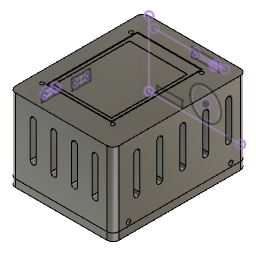
enviro-feather-box (Autodesk Fusion 360 design; units mm, degrees)
Autodesk Fusion 360 part; units mm, degrees
(part 1 of 2)
sketch "PCB" plane through (0, 0, 0) normal (0, 0, 1) x (1, 0, 0) in component "Feather HUZZAH ESP8266 v1"
  line L0 (0, 0) -> (50.8, 0)
  line L1 (50.8, 0) -> (50.8, -22.86)
  line L2 (50.8, -22.86) -> (0, -22.86)
  line L3 (0, -22.86) -> (0, 0)
  circle A0 centre (2.54, -20.32) radius 1.27
  circle A1 centre (2.54, -2.54) radius 1.27
  circle A2 centre (48.26, -21.0185) radius 1.145
  circle A3 centre (48.26, -1.905) radius 1.145
  dimension "d1_2" = 50.8
  dimension "d2_2" = 22.86
  dimension "d3_2" = 2.54
  dimension "d4_1" = 2.54
  dimension "d5_2" = 2.54
  dimension "d6_2" = 2.54
  dimension "d7_2" = 20.32
  dimension "d8_2" = 2.54
  dimension "d9_2" = 2.29
  dimension "d10_2" = 48.26
  dimension "d11_2" = 1.8415
  dimension "d12_2" = 2.29
  dimension "d13_2" = 20.955
  dimension "d14_1" = 48.26
  constraint horizontal L0
  constraint vertical L1
  constraint horizontal L2
  constraint vertical L3
  constraint coincident L0.start L3.end
  measures "d1_2" distance of L0.start L0.end
  measures "d2_2" distance of L0.start L2.end
  measures "d3_2" diameter of A0
  measures "d4_1" distance of L3 A0.centre
  measures "d5_2" distance of L2 A0.centre
  measures "d6_2" diameter of A1
  measures "d7_2" distance of L2 A1.centre
  measures "d8_2" distance of L3 A1.centre
  measures "d9_2" diameter of A2
  measures "d10_2" distance of L3 A2.centre
  measures "d11_2" distance of L2 A2.centre
  measures "d12_2" diameter of A3
  measures "d13_2" distance of L2 A3.centre
  measures "d14_1" distance of L3 A3.centre
extrude "Extrude1" add sketch "PCB" along normal blind 1.6 makes body 1 in component "Feather HUZZAH ESP8266 v1"
fillet "Fillet1" radius 2.54 4 edges at (0, -22.86, 0.8) (50.8, -22.86, 0.8) (50.8, 0, 0.8) (0, 0, 0.8) on bodies 1 in component "Feather HUZZAH ESP8266 v1"
sketch "usb" plane through (0, 0, 1.6) normal (0, 0, 1) x (-1, 0, 0) in component "Feather HUZZAH ESP8266 v1"
  circle A0 centre (-2.54, 20.32) radius 1.27
  circle A1 centre (-2.54, 2.54) radius 1.27
  circle A2 centre (-48.26, 21.0185) radius 1.145
  circle A3 centre (-48.26, 1.905) radius 1.145
  arc A4 (-2.54, 0) -> (0, 2.54) centre (-2.54, 2.54) ccw
  line L0 (0, 2.54) -> (0, 20.32)
  arc A5 (0, 20.32) -> (-2.54, 22.86) centre (-2.54, 20.32) ccw
  line L1 (-2.54, 22.86) -> (-48.26, 22.86)
  arc A6 (-48.26, 22.86) -> (-50.8, 20.32) centre (-48.26, 20.32) ccw
  line L2 (-50.8, 20.32) -> (-50.8, 2.54)
  arc A7 (-50.8, 2.54) -> (-48.26, 0) centre (-48.26, 2.54) ccw
  line L3 (-48.26, 0) -> (-2.54, 0)
  line L4 (0, 11.43) -> (-50.8, 11.43) construction
  line L5 (0, 15.33) -> (-5.6, 15.33)
  line L6 (-5.6, 15.33) -> (-5.6, 7.53)
  line L7 (-5.6, 7.53) -> (0, 7.53)
  line L8 (0, 7.53) -> (0, 15.33)
  line L9 (0, 15.33) -> (-5.6, 7.53) construction
  line L10 (-5.6, 15.33) -> (0, 7.53) construction
  point P0 (-2.8, 11.43)
  dimension "d18_1" = 7.8
  dimension "d19_1" = 5.6
  constraint midpoint L0 L4.start
  constraint midpoint L2 L4.end
  constraint perpendicular L5 L6
  constraint parallel L5 L7
  constraint parallel L6 L8
  constraint horizontal L5
  constraint coincident L9 P0
  constraint coincident L10 P0
  constraint coincident L4 P0
  constraint collinear L0 L8
  measures "d18_1" distance of L5.end L6.end
  measures "d19_1" distance of L6.end L7.end
extrude "Extrude2" add sketch "usb" along normal blind 2.95 separate body contours L0 L5 L6 L7 L8 makes body 2 in component "Feather HUZZAH ESP8266 v1"
chamfer "Chamfer1" distance 1 angle 45 2 edges at (2.8, -7.53, 1.6) (2.8, -15.33, 1.6) on bodies 2 in component "Feather HUZZAH ESP8266 v1"
sketch "modules" plane through (0, 0, 1.6) normal (0, 0, 1) x (-1, 0, 0) in component "Feather HUZZAH ESP8266 v1"
  circle A0 centre (-2.54, 20.32) radius 1.27
  circle A1 centre (-2.54, 2.54) radius 1.27
  circle A2 centre (-48.26, 21.0185) radius 1.145
  circle A3 centre (-48.26, 1.905) radius 1.145
  arc A4 (-2.54, 0) -> (0, 2.54) centre (-2.54, 2.54) ccw
  line L0 (0, 2.54) -> (0, 20.32)
  arc A5 (0, 20.32) -> (-2.54, 22.86) centre (-2.54, 20.32) ccw
  line L1 (-2.54, 22.86) -> (-48.26, 22.86)
  arc A6 (-48.26, 22.86) -> (-50.8, 20.32) centre (-48.26, 20.32) ccw
  line L2 (-50.8, 20.32) -> (-50.8, 2.54)
  arc A7 (-50.8, 2.54) -> (-48.26, 0) centre (-48.26, 2.54) ccw
  line L3 (-48.26, 0) -> (-2.54, 0)
  line L4 (-50.8, 11.43) -> (0, 11.43) construction
  line L5 (-26.8, 19.43) -> (-50.8, 19.43)
  line L6 (-50.8, 19.43) -> (-50.8, 3.43)
  line L7 (-50.8, 3.43) -> (-26.8, 3.43)
  line L8 (-26.8, 3.43) -> (-26.8, 19.43)
  line L9 (-26.8, 19.43) -> (-50.8, 3.43) construction
  line L10 (-50.8, 19.43) -> (-26.8, 3.43) construction
  line L11 (-28.4, 17.58) -> (-43.7, 17.58)
  line L12 (-43.7, 17.58) -> (-43.7, 5.28)
  line L13 (-43.7, 5.28) -> (-28.4, 5.28)
  line L14 (-28.4, 5.28) -> (-28.4, 17.58)
  line L15 (-28.4, 17.58) -> (-43.7, 5.28) construction
  line L16 (-43.7, 17.58) -> (-28.4, 5.28) construction
  point P0 (-38.8, 11.43)
  point P1 (-36.05, 11.43)
  dimension "d23_1" = 24
  dimension "d24_1" = 16
  dimension "d25_1" = 15.3
  dimension "d26_1" = 12.3
  dimension "d32_1" = 1.6
  constraint midpoint L2 L4.start
  constraint midpoint L0 L4.end
  constraint perpendicular L5 L6
  constraint parallel L5 L7
  constraint parallel L6 L8
  constraint horizontal L5
  constraint coincident L9 P0
  constraint coincident L10 P0
  constraint coincident L4 P0
  constraint perpendicular L11 L12
  constraint parallel L11 L13
  constraint parallel L12 L14
  constraint horizontal L11
  constraint coincident L15 P1
  constraint coincident L16 P1
  constraint coincident L4 P1
  measures "d23_1" distance of L6.end L7.end
  measures "d24_1" distance of L5.end L6.end
  measures "d25_1" distance of L12.end L13.end
  measures "d26_1" distance of L11.end L12.end
  measures "d32_1" distance of L8 L14
extrude "Extrude3" add sketch "modules" along normal blind 1 separate body contours L2 L5 L6 L7 L8 | L11 L12 L13 L14 makes body 3 in component "Feather HUZZAH ESP8266 v1"
extrude "Extrude4" add sketch "modules" along normal blind 2.4 and the other way blind -1 separate body contours L11 L12 L13 L14 makes body 4 in component "Feather HUZZAH ESP8266 v1"
sketch "JST" plane through (0, 0, 1.6) normal (0, 0, 1) x (-1, 0, 0) in component "Feather HUZZAH ESP8266 v1"
  circle A0 centre (-2.54, 20.32) radius 1.27
  circle A1 centre (-2.54, 2.54) radius 1.27
  circle A2 centre (-48.26, 21.0185) radius 1.145
  circle A3 centre (-48.26, 1.905) radius 1.145
  arc A4 (-2.54, 0) -> (0, 2.54) centre (-2.54, 2.54) ccw
  line L0 (0, 2.54) -> (0, 20.32)
  arc A5 (0, 20.32) -> (-2.54, 22.86) centre (-2.54, 20.32) ccw
  line L1 (-2.54, 22.86) -> (-48.26, 22.86)
  arc A6 (-48.26, 22.86) -> (-50.8, 20.32) centre (-48.26, 20.32) ccw
  line L2 (-50.8, 20.32) -> (-50.8, 2.54)
  arc A7 (-50.8, 2.54) -> (-48.26, 0) centre (-48.26, 2.54) ccw
  line L3 (-48.26, 0) -> (-2.54, 0)
  line L4 (-6.8, 0) -> (-14.8, 0)
  line L5 (-14.8, 0) -> (-14.8, 6)
  line L6 (-14.8, 6) -> (-6.8, 6)
  line L7 (-6.8, 6) -> (-6.8, 0)
  line L8 (-10.8, 0) -> (-10.8, 6) construction
  dimension "d33_1" = 8
  dimension "d34_1" = 6
  dimension "d35_1" = 10.8
  constraint horizontal L4
  constraint vertical L5
  constraint horizontal L6
  constraint vertical L7
  constraint midpoint L4 L8.start
  constraint midpoint L6 L8.end
  constraint collinear L3 L4
  measures "d33_1" distance of L4.start L4.end
  measures "d34_1" distance of L4.start L6.end
  measures "d35_1" distance of L0 L8
extrude "Extrude5" add sketch "JST" along normal blind 5.6 separate body contours L3 L4 L5 L6 L7 makes body 5 in component "Feather HUZZAH ESP8266 v1"
sketch "headers" plane through (0, 0, 1.6) normal (0, 0, 1) x (-1, 0, 0) in component "Feather HUZZAH ESP8266 v1"
  circle A0 centre (-48.26, 21.0185) radius 1.145
  circle A1 centre (-2.54, 2.54) radius 1.27
  circle A2 centre (-48.26, 1.905) radius 1.145
  circle A3 centre (-2.54, 20.32) radius 1.27
  arc A4 (-2.54, 0) -> (0, 2.54) centre (-2.54, 2.54) ccw
  line L0 (0, 2.54) -> (0, 20.32)
  arc A5 (0, 20.32) -> (-2.54, 22.86) centre (-2.54, 20.32) ccw
  line L1 (-2.54, 22.86) -> (-48.26, 22.86)
  arc A6 (-48.26, 22.86) -> (-50.8, 20.32) centre (-48.26, 20.32) ccw
  line L2 (-50.8, 20.32) -> (-50.8, 2.54)
  arc A7 (-50.8, 2.54) -> (-48.26, 0) centre (-48.26, 2.54) ccw
  line L3 (-48.26, 0) -> (-2.54, 0)
  line L4 (-15, 0) -> (-45.8, 0)
  line L5 (-45.8, 0) -> (-45.8, 2.6)
  line L6 (-45.8, 2.6) -> (-15, 2.6)
  line L7 (-15, 2.6) -> (-15, 0)
  line L8 (-6.2, 20.36) -> (-44.8, 20.36)
  line L9 (-44.8, 20.36) -> (-44.8, 22.86)
  line L10 (-44.8, 22.86) -> (-6.2, 22.86)
  line L11 (-6.2, 22.86) -> (-6.2, 20.36)
  dimension "d39_1" = 30.8
  dimension "d40_1" = 2.6
  dimension "d42_1" = 5
  dimension "d45_1" = 38.6
  dimension "d46_1" = 2.5
  dimension "d48_1" = 6
  constraint horizontal L4
  constraint vertical L5
  constraint horizontal L6
  constraint vertical L7
  constraint horizontal L8
  constraint vertical L9
  constraint horizontal L10
  constraint vertical L11
  constraint collinear L3 L4
  constraint collinear L1 L10
  measures "d39_1" distance of L4.start L4.end
  measures "d40_1" distance of L4.start L6.end
  measures "d42_1" distance of L2 L5
  measures "d45_1" distance of L8.start L8.end
  measures "d46_1" distance of L8.start L10.end
  measures "d48_1" distance of L2 L9
extrude "Extrude6" add sketch "headers" along normal blind 2.5 separate body contours L3 L4 L5 L6 L7 | L1 L8 L9 L10 L11 makes body 6 at (25.2667, -1.7333, 1.6) makes body 7 at (31.9333, -22.0267, 1.6) in component "Feather HUZZAH ESP8266 v1"
move_body "Move1" bodies 7 6 to x (1, 0, 0) y (0, 1, 0) z (0, 0, 1) at (0, 0, -4.1) in component "Feather HUZZAH ESP8266 v1"
sketch "pcb" plane through (0, 0, 0) normal (0, 0, 1) x (1, 0, 0) in component "2.4\" TFT Feather Wing Copy v1"
  line L0 (0, 0) -> (64.77, 0)
  line L1 (64.77, 0) -> (64.77, 52.578)
  line L2 (64.77, 52.578) -> (0, 52.578)
  line L3 (0, 52.578) -> (0, 0)
  circle A0 centre (2.54, 50.038) radius 1.27
  line L4 (32.385, 52.578) -> (32.385, 0) construction
  line L5 (0, 26.289) -> (64.77, 26.289) construction
  circle A1 centre (62.23, 50.038) radius 1.27
  circle A2 centre (2.54, 2.54) radius 1.27
  circle A3 centre (62.23, 2.54) radius 1.27
  dimension "d1_1" = 64.77
  dimension "d2_1" = 52.578
  dimension "d3_1" = 2.54
  dimension "d4" = 2.54
  dimension "d5_1" = 2.54
  constraint horizontal L0
  constraint vertical L1
  constraint horizontal L2
  constraint vertical L3
  constraint coincident L0.start L3.end
  constraint midpoint L2 L4.start
  constraint midpoint L0 L4.end
  constraint midpoint L3 L5.start
  constraint midpoint L1 L5.end
  constraint symmetric A0 L4 A1
  constraint symmetric A0 L5 A2
  constraint symmetric L5 A1 A3
  measures "d1_1" distance of L1.end L2.end
  measures "d2_1" distance of L0.start L2.end
  measures "d3_1" diameter of A0
  measures "d4" distance of L3 A0.centre
  measures "d5_1" distance of L2 A0.centre
extrude "Extrude1'" add sketch "pcb" along normal blind 1.6 separate body makes body 8 in component "2.4\" TFT Feather Wing Copy v1"
fillet "Fillet1'" radius 2.54 4 edges at (64.77, 0, 0.8) (0, 0, 0.8) (0, 52.578, 0.8) (64.77, 52.578, 0.8) on bodies 8 in component "2.4\" TFT Feather Wing Copy v1"
sketch "bottom" plane through (0, 0, 0) normal (0, 0, -1) x (1, 0, 0) in component "2.4\" TFT Feather Wing Copy v1"
  circle A0 centre (62.23, -50.038) radius 1.27
  circle A1 centre (2.54, -2.54) radius 1.27
  circle A2 centre (62.23, -2.54) radius 1.27
  circle A3 centre (2.54, -50.038) radius 1.27
  arc A4 (62.23, -52.578) -> (64.77, -50.038) centre (62.23, -50.038) ccw
  line L0 (64.77, -50.038) -> (64.77, -2.54)
  arc A5 (64.77, -2.54) -> (62.23, 0) centre (62.23, -2.54) ccw
  line L1 (62.23, 0) -> (2.54, 0)
  arc A6 (2.54, 0) -> (0, -2.54) centre (2.54, -2.54) ccw
  line L2 (0, -2.54) -> (0, -50.038)
  arc A7 (0, -50.038) -> (2.54, -52.578) centre (2.54, -50.038) ccw
  line L3 (2.54, -52.578) -> (62.23, -52.578)
  line L4 (62.97, -45.978) -> (57.97, -45.978)
  line L5 (57.97, -45.978) -> (57.97, -14.978)
  line L6 (57.97, -14.978) -> (62.97, -14.978)
  line L7 (62.97, -14.978) -> (62.97, -45.978)
  line L8 (40.17, -45.978) -> (35.17, -45.978)
  line L9 (35.17, -45.978) -> (35.17, -4.978)
  line L10 (35.17, -4.978) -> (40.17, -4.978)
  line L11 (40.17, -4.978) -> (40.17, -45.978)
  line L12 (1.6, -6.8) -> (7.6, -6.8)
  line L13 (7.6, -6.8) -> (7.6, -12.8)
  line L14 (7.6, -12.8) -> (1.6, -12.8)
  line L15 (1.6, -12.8) -> (1.6, -6.8)
  line L16 (1.6, -6.8) -> (7.6, -12.8) construction
  line L17 (7.6, -6.8) -> (1.6, -12.8) construction
  circle A8 centre (4.6, -9.8) radius 1.5
  line L18 (5.5, -17.4) -> (2, -17.4)
  line L19 (2, -17.4) -> (2, -24.4)
  line L20 (2, -24.4) -> (5.5, -24.4)
  line L21 (5.5, -24.4) -> (5.5, -17.4)
  line L22 (15.5, -43.978) -> (0, -43.978)
  line L23 (0, -43.978) -> (0, -29.978)
  line L24 (0, -29.978) -> (15.5, -29.978)
  line L25 (15.5, -29.978) -> (15.5, -43.978)
  point P0 (4.6, -9.8)
  dimension "d9_1" = 5
  dimension "d10_1" = 5
  dimension "d11_1" = 31
  dimension "d12_1" = 41
  dimension "d13_1" = 6.6
  dimension "d14" = 6.6
  dimension "d15" = 1.8
  dimension "d16" = 17.8
  dimension "d19" = 6
  dimension "d20" = 6
  dimension "d21" = 6.8
  dimension "d22" = 1.6
  dimension "d23" = 3
  dimension "d28" = 3.5
  dimension "d29" = 7
  dimension "d30" = 2
  dimension "d31" = 17.4
  dimension "d32" = 15.5
  dimension "d33" = 14
  dimension "d34" = 8.6
  constraint horizontal L4
  constraint vertical L5
  constraint horizontal L6
  constraint vertical L7
  constraint horizontal L8
  constraint vertical L9
  constraint horizontal L10
  constraint vertical L11
  constraint perpendicular L12 L13
  constraint parallel L12 L14
  constraint parallel L13 L15
  constraint horizontal L12
  constraint coincident L16 P0
  constraint coincident L17 P0
  constraint coincident P0 A8.centre
  constraint horizontal L18
  constraint vertical L19
  constraint horizontal L20
  constraint vertical L21
  constraint horizontal L22
  constraint vertical L23
  constraint horizontal L24
  constraint vertical L25
  constraint collinear L2 L23
  measures "d9_1" distance of L5.end L6.end
  measures "d10_1" distance of L9.end L10.end
  measures "d11_1" distance of L4.start L6.end
  measures "d12_1" distance of L8.start L10.end
  measures "d13_1" distance of L3 L4
  measures "d14" distance of L3 L8
  measures "d15" distance of L0 L7
  measures "d16" distance of L5 L11
  measures "d19" distance of L13.end L14.end
  measures "d20" distance of L12.end L13.end
  measures "d21" distance of L1 L12
  measures "d22" distance of L2 L15
  measures "d23" diameter of A8
  measures "d28" distance of L18.start L18.end
  measures "d29" distance of L18.start L20.end
  measures "d30" distance of L2 L19
  measures "d31" distance of L1 L18
  measures "d32" distance of L22.start L22.end
  measures "d33" distance of L22.start L24.end
  measures "d34" distance of L3 L22
extrude "Extrude2'" add sketch "bottom" along normal blind 3.9 separate body contours L4 L5 L6 L7 | L8 L9 L10 L11 makes body 9 at (61.3033, 25.3113, 0) makes body 10 at (38.5033, 32.3113, 0) in component "2.4\" TFT Feather Wing Copy v1"
extrude "Extrude3'" add sketch "bottom" along normal blind 1.8 separate body contours L12 L13 L14 L15 | A8 makes body 11 in component "2.4\" TFT Feather Wing Copy v1"
extrude "Extrude4'" add sketch "bottom" along normal blind 3 contours A8 bodies 11 in component "2.4\" TFT Feather Wing Copy v1"
extrude "Extrude5'" add sketch "bottom" along normal blind 1.4 separate body contours L18 L19 L20 L21 makes body 12 in component "2.4\" TFT Feather Wing Copy v1"
extrude "Extrude6'" add sketch "bottom" along normal blind 1.7 separate body contours L2 L22 L23 L24 L25 makes body 13 in component "2.4\" TFT Feather Wing Copy v1"
sketch "microSD" plane through (0, 0, -1.7) normal (0, 0, -1) x (1, 0, 0) in component "2.4\" TFT Feather Wing Copy v1"
  line L0 (15.5, -29.978) -> (0, -29.978)
  line L1 (0, -29.978) -> (0, -43.978)
  line L2 (0, -43.978) -> (15.5, -43.978)
  line L3 (15.5, -43.978) -> (15.5, -29.978)
  circle A0 centre (-8.5, -35.5) radius 11
  dimension "d39" = 22
  measures "d39" diameter of A0
extrude "Extrude7" cut sketch "microSD" against normal blind 1.7 contours L0 L1 A0 picked at (0.2923, -37.9037) bodies 13 in component "2.4\" TFT Feather Wing Copy v1"
sketch "switch" plane through (0, 0, -1.4) normal (0, 0, -1) x (1, 0, 0) in component "2.4\" TFT Feather Wing Copy v1"
  line L0 (5.5, -24.4) -> (5.5, -17.4)
  line L1 (5.5, -17.4) -> (2, -17.4)
  line L2 (2, -17.4) -> (2, -24.4)
  line L3 (2, -24.4) -> (5.5, -24.4)
  line L4 (2, -20.9) -> (5.5, -20.9)
  line L5 (2, -19.4) -> (3, -19.4)
  line L6 (3, -19.4) -> (3, -22.4)
  line L7 (3, -22.4) -> (2, -22.4)
  line L8 (2, -22.4) -> (2, -19.4)
  line L9 (3, -20.9) -> (2, -20.9) construction
  dimension "d42" = 3
  dimension "d43" = 1
  constraint midpoint L2 L4.start
  constraint midpoint L0 L4.end
  constraint horizontal L5
  constraint vertical L6
  constraint horizontal L7
  constraint vertical L8
  constraint coincident L2 L5.start
  constraint midpoint L6 L9.start
  constraint midpoint L8 L4.start
  constraint collinear L4 L9
  measures "d42" distance of L5.end L6.end
  measures "d43" distance of L6.end L7.end
extrude "Extrude8" add sketch "switch" along normal blind 1 contours L2 L4 L6 L7 L8 bodies 12 in component "2.4\" TFT Feather Wing Copy v1"
sketch "display" plane through (0, 0, 1.6) normal (0, 0, 1) x (-1, 0, 0) in component "2.4\" TFT Feather Wing Copy v1"
  arc A0 (-64.77, -50.038) -> (-62.23, -52.578) centre (-62.23, -50.038) ccw
  line L0 (-62.23, -52.578) -> (-2.54, -52.578)
  arc A1 (-2.54, -52.578) -> (0, -50.038) centre (-2.54, -50.038) ccw
  line L1 (0, -50.038) -> (0, -2.54)
  arc A2 (0, -2.54) -> (-2.54, 0) centre (-2.54, -2.54) ccw
  line L2 (-2.54, 0) -> (-62.23, 0)
  arc A3 (-62.23, 0) -> (-64.77, -2.54) centre (-62.23, -2.54) ccw
  line L3 (-64.77, -2.54) -> (-64.77, -50.038)
  circle A4 centre (-62.23, -50.038) radius 1.27
  circle A5 centre (-2.54, -2.54) radius 1.27
  circle A6 centre (-62.23, -2.54) radius 1.27
  circle A7 centre (-2.54, -50.038) radius 1.27
  line L4 (-0.8, -47.778) -> (-61, -47.778)
  line L5 (-61, -47.778) -> (-61, -4.978)
  line L6 (-61, -4.978) -> (-0.8, -4.978)
  line L7 (-0.8, -4.978) -> (-0.8, -47.778)
  dimension "d46" = 60.2
  dimension "d47" = 42.8
  dimension "d48" = 4.8
  dimension "d49" = 0.8
  constraint horizontal L4
  constraint vertical L5
  constraint horizontal L6
  constraint vertical L7
  measures "d46" distance of L4.start L4.end
  measures "d47" distance of L4.start L6.end
  measures "d48" distance of L0 L4
  measures "d49" distance of L1 L7
extrude "Extrude9" add sketch "display" along normal blind 3.9 separate body contours L4 L5 L6 L7 makes body 14 in component "2.4\" TFT Feather Wing Copy v1"
sketch "view" plane through (0, 0, 5.5) normal (0, 0, 1) x (-1, 0, 0) in component "2.4\" TFT Feather Wing Copy v1"
  line L0 (-0.8, -4.978) -> (-61, -4.978)
  line L1 (-61, -4.978) -> (-61, -47.778)
  line L2 (-61, -47.778) -> (-0.8, -47.778)
  line L3 (-0.8, -47.778) -> (-0.8, -4.978)
  line L4 (-8, -45.778) -> (-59, -45.778)
  line L5 (-59, -45.778) -> (-59, -6.978)
  line L6 (-59, -6.978) -> (-8, -6.978)
  line L7 (-8, -6.978) -> (-8, -45.778)
  dimension "d52" = 2
  dimension "d53" = 2
  dimension "d54" = 2
  dimension "d55" = 7.2
  constraint horizontal L4
  constraint vertical L5
  constraint horizontal L6
  constraint vertical L7
  measures "d52" distance of L0 L6
  measures "d53" distance of L1 L5
  measures "d54" distance of L2 L4
  measures "d55" distance of L3 L7
extrude "Extrude10" cut sketch "view" against normal blind 0.2 contours L4 L5 L6 L7 bodies 14 in component "2.4\" TFT Feather Wing Copy v1"
sketch "Sketch6" plane through (0, 0, 1.6) normal (0, 0, 1) x (-1, 0, 0) in component "Feather HUZZAH ESP8266 v1"
  circle A0 centre (-2.54, 20.32) radius 1.27
  circle A1 centre (-2.54, 2.54) radius 1.27
  circle A2 centre (-48.26, 21.0185) radius 1.145
  circle A3 centre (-48.26, 1.905) radius 1.145
  arc A4 (-2.54, 0) -> (0, 2.54) centre (-2.54, 2.54) ccw
  line L0 (0, 2.54) -> (0, 20.32)
  arc A5 (0, 20.32) -> (-2.54, 22.86) centre (-2.54, 20.32) ccw
  line L1 (-2.54, 22.86) -> (-48.26, 22.86)
  arc A6 (-48.26, 22.86) -> (-50.8, 20.32) centre (-48.26, 20.32) ccw
  line L2 (-50.8, 20.32) -> (-50.8, 2.54)
  arc A7 (-50.8, 2.54) -> (-48.26, 0) centre (-48.26, 2.54) ccw
  line L3 (-48.26, 0) -> (-2.54, 0)
  line L4 (-4.8, 20.41) -> (-46, 20.41)
  line L5 (-46, 20.41) -> (-46, 22.86)
  line L6 (-46, 22.86) -> (-4.8, 22.86)
  line L7 (-4.8, 22.86) -> (-4.8, 20.41)
  line L8 (-25.4, 0) -> (-25.4, 16) construction
  line L9 (-25.4, 20.41) -> (-25.4, 22.86) construction
  line L10 (-15.9, 0) -> (-46, 0)
  line L11 (-46, 0) -> (-46, 2.45)
  line L12 (-46, 2.45) -> (-15.9, 2.45)
  line L13 (-15.9, 2.45) -> (-15.9, 0)
  dimension "d79" = 41.2
  dimension "d80" = 2.45
  dimension "d81" = 30.1
  constraint horizontal L4
  constraint vertical L5
  constraint horizontal L6
  constraint vertical L7
  constraint collinear L1 L6
  constraint midpoint L3 L8.start
  constraint perpendicular L4 L8
  constraint midpoint L4 L9.start
  constraint midpoint L6 L9.end
  constraint collinear L8 L9
  constraint horizontal L10
  constraint vertical L11
  constraint horizontal L12
  constraint vertical L13
  constraint equal L5 L11
  constraint collinear L3 L10
  measures "d79" distance of L4.start L4.end
  measures "d80" distance of L4.start L6.end
  measures "d81" distance of L10.start L10.end
extrude "Extrude7'" add sketch "Sketch6" along normal blind 8.6 contours L3 L10 L11 L12 L13 | L1 L4 L5 L6 L7 bodies 1 in component "Feather HUZZAH ESP8266 v1"
sketch "Sketch1" plane through (0, 0, 30.3885) normal (0, 0, -1) x (1, 0, 0) in component "sensors"
  line L0 (24.8533, -55.1266) -> (24.8533, -57.5766)
  line L1 (24.8533, -57.5766) -> (27.1133, -57.5766)
  arc A0 (27.1133, -57.5766) -> (29.6533, -55.0366) centre (27.1133, -55.0366) ccw
  line L2 (29.6533, -55.0366) -> (29.6533, -37.2566)
  arc A1 (29.6533, -37.2566) -> (27.1133, -34.7166) centre (27.1133, -37.2566) ccw
  line L3 (27.1133, -34.7166) -> (24.8533, -34.7166)
  line L4 (24.8533, -34.7166) -> (24.8533, -37.1666)
  line L5 (24.8533, -37.1666) -> (-5.2467, -37.1666)
  line L6 (-5.2467, -37.1666) -> (-5.2467, -34.7166)
  line L7 (-5.2467, -34.7166) -> (-18.6067, -34.7166)
  arc A2 (-18.6067, -34.7166) -> (-21.1467, -37.2566) centre (-18.6067, -37.2566) ccw
  line L8 (-21.1467, -37.2566) -> (-21.1467, -55.0366)
  arc A3 (-21.1467, -55.0366) -> (-18.6067, -57.5766) centre (-18.6067, -55.0366) ccw
  line L9 (-18.6067, -57.5766) -> (-16.3467, -57.5766)
  line L10 (-16.3467, -57.5766) -> (-16.3467, -55.1266)
  line L11 (-16.3467, -55.1266) -> (24.8533, -55.1266)
  circle A4 centre (27.1133, -36.6216) radius 1.145
  circle A5 centre (27.1133, -55.7351) radius 1.145
  circle A6 centre (-18.6067, -37.2566) radius 1.27
  circle A7 centre (-18.6067, -55.0366) radius 1.27
  line L12 (-5.2467, -34.7166) -> (24.8533, -34.7166)
  line L13 (24.8533, -34.7166) -> (24.8533, -37.1666)
  line L14 (24.8533, -37.1666) -> (-5.2467, -37.1666)
  line L15 (-5.2467, -37.1666) -> (-5.2467, -34.7166)
  line L16 (24.8533, -55.1266) -> (-16.3467, -55.1266)
  line L17 (-16.3467, -55.1266) -> (-16.3467, -57.5766)
  line L18 (-16.3467, -57.5766) -> (24.8533, -57.5766)
  line L19 (24.8533, -57.5766) -> (24.8533, -55.1266)
  constraint horizontal L12
  constraint vertical L13
  constraint horizontal L14
  constraint vertical L15
  constraint coincident L4.end L5.start
  constraint coincident L6.end L7.start
  constraint horizontal L16
  constraint vertical L17
  constraint horizontal L18
  constraint vertical L19
  constraint coincident L9.end L10.start
  constraint coincident L0.start L11.end
extrude "Extrude1''" add sketch "Sketch1" along normal blind 1.66 separate body contours L0 L1 A0 L2 A1 L3 L4 L5 L6 L7 A2 L8 A3 L9 L10 L11 L13 L14 L15 L16 L17 L19 makes body 15 in component "sensors"
extrude "Extrude2''" add sketch "Sketch1" along normal blind 1.66 and the other way blind 2.66 contours L0 L10 L11 L16 L17 L18 L19 | L4 L5 L6 L12 L13 L14 L15 bodies 15 in component "sensors"
sketch "Sketch1 (2)" plane through (0, 0, 0) normal (0, 0, 1) x (1, 0, 0) in component "pms5003"
  line L0 (0, 0) -> (50.1, 0)
  line L1 (50.1, 0) -> (50.1, -38.2)
  line L2 (50.1, -38.2) -> (0, -38.2)
  line L3 (0, -38.2) -> (0, 0)
  dimension "d98" = 50.1
  dimension "d99" = 38.2
  constraint horizontal L0
  constraint vertical L1
  constraint horizontal L2
  constraint vertical L3
  constraint coincident L0.start L3.end
  measures "d98" distance of L0.start L0.end
  measures "d99" distance of L0.end L1.end
extrude "Extrude1'''" add sketch "Sketch1 (2)" along normal blind 21.3 separate body makes body 16 in component "pms5003"
fillet "Fillet1''" radius 1 4 edges at (50.1, 0, 10.65) (50.1, -38.2, 10.65) (0, 0, 10.65) (0, -38.2, 10.65) on bodies 16 in component "pms5003"
sketch "Sketch2" plane through (0, 0, 0) normal (0, 1, 0) x (-1, 0, 0) in component "pms5003"
  line L0 (-1, 0) -> (-1, 21.3)
  line L1 (-1, 21.3) -> (-49.1, 21.3)
  line L2 (-49.1, 21.3) -> (-49.1, 0)
  line L3 (-49.1, 0) -> (-1, 0)
  circle A0 centre (-36.1, 10.65) radius 9
  circle A1 centre (-18, 2.5) radius 1.25
  line L4 (-49.1, 10.65) -> (-1, 10.65) construction
  line L5 (-50.1, 21.3) -> (-50.1, 0) construction
  line L6 (0, 0) -> (0, 21.3) construction
  circle A2 centre (-14, 2.5) radius 1.25
  circle A3 centre (-10, 2.5) radius 1.25
  circle A4 centre (-6, 2.5) radius 1.25
  dimension "d104" = 18
  dimension "d105" = 14
  dimension "d106" = 2.5
  dimension "d107" = 18
  dimension "d108" = 2.5
  dimension "d111" = 12
  dimension "d112" = 0
  constraint midpoint L2 L4.start
  constraint midpoint L0 L4.end
  constraint coincident A0.centre L4
  measures "d104" diameter of A0
  measures "d105" distance of A0.centre L5
  measures "d106" diameter of A1
  measures "d107" distance of A1.centre L6
  measures "d108" distance of L3 A1.centre
extrude "Extrude2'''" cut sketch "Sketch2" against normal blind 4 contours A0 | A1 | A2 | A3 | A4 bodies 16 in component "pms5003"
sketch "Sketch3" plane through (0, -38.2, 0) normal (0, -1, 0) x (1, 0, 0) in component "pms5003"
  line L0 (1, 21.3) -> (1, 0)
  line L1 (1, 0) -> (49.1, 0)
  line L2 (49.1, 0) -> (49.1, 21.3)
  line L3 (49.1, 21.3) -> (1, 21.3)
  line L4 (27.3, 13.225) -> (44.6, 13.225)
  line L5 (44.6, 13.225) -> (44.6, 8.075)
  line L6 (44.6, 8.075) -> (27.3, 8.075)
  line L7 (27.3, 8.075) -> (27.3, 13.225)
  line L8 (1, 10.65) -> (50, 10.65) construction
  line L9 (50.1, 0) -> (50.1, 21.3) construction
  dimension "d115" = 17.3
  dimension "d116" = 5.15
  dimension "d117" = 5.5
  dimension "d118" = 2.575
  constraint horizontal L4
  constraint vertical L5
  constraint horizontal L6
  constraint vertical L7
  constraint midpoint L0 L8.start
  constraint perpendicular L0 L8
  measures "d115" distance of L4.start L4.end
  measures "d116" distance of L4.start L6.end
  measures "d117" distance of L5 L9
  measures "d118" distance of L4 L8
extrude "Extrude3''" cut sketch "Sketch3" against normal blind 3 contours L4 L5 L6 L7 bodies 16 in component "pms5003"
sketch "Sketch1 (3)" plane through (0, 0, 21.3) normal (0, 0, 1) x (-1, 0, 0) in component "jlink"
  arc A0 (0, 37.2) -> (-1, 38.2) centre (-1, 37.2) ccw
  line L0 (-1, 38.2) -> (-49.1, 38.2)
  arc A1 (-49.1, 38.2) -> (-50.1, 37.2) centre (-49.1, 37.2) ccw
  line L1 (-50.1, 37.2) -> (-50.1, 1)
  arc A2 (-50.1, 1) -> (-49.1, 0) centre (-49.1, 1) ccw
  line L2 (-49.1, 0) -> (-1, 0)
  arc A3 (-1, 0) -> (0, 1) centre (-1, 1) ccw
  line L3 (0, 1) -> (0, 37.2)
  line L4 (0, 0) -> (-34.7, 0)
  line L5 (-34.7, 0) -> (-34.7, 17.2)
  line L6 (-34.7, 17.2) -> (0, 17.2)
  line L7 (0, 17.2) -> (0, 0)
  line L8 (-34.7, 1.35) -> (-27.7, 1.35)
  line L9 (-27.7, 1.35) -> (-27.7, 15.85) construction
  line L10 (-27.7, 15.85) -> (-34.7, 15.85)
  line L11 (-34.7, 15.85) -> (-34.7, 1.35)
  line L12 (0, 1) -> (-3.3, 1)
  line L13 (-3.3, 1) -> (-3.3, 16.2) construction
  line L14 (-3.3, 16.2) -> (0, 16.2)
  line L15 (0, 16.2) -> (0, 1) construction
  line L16 (-27.7, 1.35) -> (-27.7, 0)
  line L17 (-27.7, 15.85) -> (-27.7, 17.2)
  line L18 (-3.3, 16.2) -> (-3.3, 17.2)
  line L19 (-3.3, 1) -> (-3.3, 0)
  dimension "d121" = 34.7
  dimension "d122" = 17.2
  dimension "d123" = 14.5
  dimension "d124" = 7
  dimension "d125" = 3.3
  dimension "d126" = 15.2
  constraint horizontal L4
  constraint vertical L5
  constraint horizontal L6
  constraint vertical L7
  constraint horizontal L8
  constraint vertical L9
  constraint horizontal L10
  constraint vertical L11
  constraint coincident L5 L8.start
  constraint horizontal L12
  constraint vertical L13
  constraint horizontal L14
  constraint vertical L15
  constraint coincident L7 A3.end
  constraint coincident L4 L16.end
  constraint perpendicular L4 L16
  constraint coincident L6 L17.end
  constraint perpendicular L6 L17
  constraint coincident L6 L18.end
  constraint perpendicular L6 L18
  constraint coincident L4 L19.end
  constraint perpendicular L4 L19
  constraint equal L16 L17
  constraint equal L18 L19
  constraint coincident L4.start L7.end
  measures "d121" distance of L4.start L4.end
  measures "d122" distance of L4.start L6.end
  measures "d123" distance of L8.end L9.end
  measures "d124" distance of L8.start L8.end
  measures "d125" distance of A3.end L12.end
  measures "d126" distance of L12.end L13.end
extrude "Extrude1''''" add sketch "Sketch1 (3)" along normal blind 1.66 separate body contours L2 L3 L4 L5 L6 L7 L8 L10 L11 L12 L14 L16 L17 L18 L19 makes body 17 in component "jlink"
sketch "Sketch2 (2)" plane through (0, 0, 22.96) normal (0, 0, 1) x (-1, 0, 0) in component "jlink"
  line L0 (-3.3, 16.2) -> (-3.3, 17.2)
  line L1 (-3.3, 17.2) -> (-27.7, 17.2)
  line L2 (-27.7, 17.2) -> (-27.7, 15.85)
  line L3 (-27.7, 15.85) -> (-34.7, 15.85)
  line L4 (-34.7, 15.85) -> (-34.7, 1.35)
  line L5 (-34.7, 1.35) -> (-27.7, 1.35)
  line L6 (-27.7, 1.35) -> (-27.7, 0)
  line L7 (-27.7, 0) -> (-3.3, 0)
  line L8 (-3.3, 0) -> (-3.3, 1)
  line L9 (-3.3, 1) -> (0, 1)
  line L10 (0, 1) -> (0, 16.2)
  line L11 (0, 16.2) -> (-3.3, 16.2)
  line L12 (-27.1, 3.25) -> (-30.2, 3.25)
  line L13 (-30.2, 3.25) -> (-30.2, 13.95)
  line L14 (-30.2, 13.95) -> (-27.1, 13.95)
  line L15 (-27.1, 13.95) -> (-27.1, 3.25)
  line L16 (-34.7, 8.6) -> (0, 8.6) construction
  line L17 (-27.1, 8.6) -> (-30.2, 8.6) construction
  line L18 (-4.5, 4.6) -> (1.5, 4.6)
  line L19 (1.5, 4.6) -> (1.5, 12.6)
  line L20 (1.5, 12.6) -> (-4.5, 12.6)
  line L21 (-4.5, 12.6) -> (-4.5, 4.6)
  line L22 (1.5, 8.6) -> (-4.5, 8.6) construction
  dimension "d129" = 10.7
  dimension "d130" = 3.1
  dimension "d131" = 4.5
  dimension "d134" = 8
  dimension "d135" = 6
  dimension "d136" = 4.5
  constraint horizontal L12
  constraint vertical L13
  constraint horizontal L14
  constraint vertical L15
  constraint midpoint L4 L16.start
  constraint midpoint L10 L16.end
  constraint midpoint L15 L17.start
  constraint midpoint L13 L17.end
  constraint collinear L16 L17
  constraint horizontal L18
  constraint vertical L19
  constraint horizontal L20
  constraint vertical L21
  constraint midpoint L19 L22.start
  constraint midpoint L21 L22.end
  constraint collinear L16 L22
  measures "d129" distance of L12.start L14.end
  measures "d130" distance of L12.start L12.end
  measures "d131" distance of L4 L13
  measures "d134" distance of L18.end L19.end
  measures "d135" distance of L18.start L18.end
  measures "d136" distance of L10 L21
extrude "Extrude3'''" add sketch "Sketch2 (2)" along normal blind 3 contours L10 L18 L19 L20 | L10 L18 L20 L21 bodies 17 in component "jlink"
extrude "Extrude2''''" add sketch "Sketch2 (2)" along normal blind 8.1 contours L12 L13 L14 L15 bodies 17 in component "jlink"
sketch "Sketch1 (4)" plane through (0, 0, 38.3885) normal (0, 0, -1) x (1, 0, 0) in component "screen-pms5003-joint"
  circle A0 centre (28.8133, -33.0566) radius 1.27
  circle A1 centre (-18.6847, -92.7466) radius 1.27
  circle A2 centre (28.8133, -92.7466) radius 1.27
  circle A3 centre (-18.6847, -33.0566) radius 1.27
  arc A4 (31.3533, -33.0566) -> (28.8133, -30.5166) centre (28.8133, -33.0566) ccw
  line L0 (28.8133, -30.5166) -> (-18.6847, -30.5166)
  arc A5 (-18.6847, -30.5166) -> (-21.2247, -33.0566) centre (-18.6847, -33.0566) ccw
  line L1 (-21.2247, -33.0566) -> (-21.2247, -92.7466)
  arc A6 (-21.2247, -92.7466) -> (-18.6847, -95.2866) centre (-18.6847, -92.7466) ccw
  line L2 (-18.6847, -95.2866) -> (28.8133, -95.2866)
  arc A7 (28.8133, -95.2866) -> (31.3533, -92.7466) centre (28.8133, -92.7466) ccw
  line L3 (31.3533, -92.7466) -> (31.3533, -33.0566)
  line L4 (-21.2247, -76.2866) -> (-16.2467, -76.2866)
  line L5 (-16.2467, -76.2866) -> (-16.2467, -95.2866)
  line L6 (-16.2467, -95.2866) -> (-21.2247, -95.2866)
  line L7 (-21.2247, -95.2866) -> (-21.2247, -76.2866)
  line L8 (-16.2467, -34.2866) -> (-16.2467, -94.4866)
  line L9 (5.0643, -30.5166) -> (5.0643, -95.2866) construction
  line L10 (26.3753, -76.2866) -> (26.3753, -95.2866)
  line L11 (26.3753, -95.2866) -> (31.3533, -95.2866)
  line L12 (31.3533, -76.2866) -> (26.3753, -76.2866)
  line L13 (31.3533, -95.2866) -> (31.3533, -76.2866)
  dimension "d143" = 19
  constraint horizontal L4
  constraint vertical L5
  constraint horizontal L6
  constraint vertical L7
  constraint coincident L2 L5.end
  constraint coincident L1 L4.start
  constraint coincident L4.end L8
  constraint midpoint L0 L9.start
  constraint midpoint L2 L9.end
  constraint symmetric L4.start L9 L12.start
  constraint symmetric L4.end L9 L10.start
  constraint symmetric L5.end L9 L10.end
  constraint symmetric L6.end L9 L11.end
  measures "d143" distance of L4.start L6.end
extrude "Extrude1'''''" add sketch "Sketch1 (4)" along normal blind 4 separate body contours L2 A7 L3 L10 L11 L12 L13 | L1 A6 L2 L4 L5 L6 L7 L8 makes body 18 at (28.8789, 81.3511, 38.3885) makes body 19 at (-18.7504, 81.3511, 38.3885) in component "screen-pms5003-joint"
sketch "Sketch2 (3)" plane through (0, 0, 34.3885) normal (0, 0, -1) x (1, 0, 0) in component "screen-pms5003-joint"
  circle A0 centre (-18.6847, -92.7466) radius 1.27
  arc A1 (-21.2247, -92.7466) -> (-18.6847, -95.2866) centre (-18.6847, -92.7466) ccw
  line L0 (-18.6847, -95.2866) -> (-16.2467, -95.2866)
  line L1 (-16.2467, -95.2866) -> (-16.2467, -76.2866)
  line L2 (-16.2467, -76.2866) -> (-21.2247, -76.2866)
  line L3 (-21.2247, -76.2866) -> (-21.2247, -92.7466)
  line L4 (-21.2247, -76.2866) -> (31.3533, -76.2866)
  line L5 (31.3533, -76.2866) -> (31.3533, -95.2866)
  line L6 (31.3533, -95.2866) -> (-21.2247, -95.2866)
  line L7 (-21.2247, -95.2866) -> (-21.2247, -76.2866)
  line L8 (31.3533, -92.7466) -> (31.3533, -76.2866)
  line L9 (28.8133, -95.2866) -> (-18.6847, -95.2866)
  constraint horizontal L4
  constraint vertical L5
  constraint horizontal L6
  constraint vertical L7
  constraint coincident L2.end L3.start
  constraint collinear L5 L8
  constraint collinear L6 L9
extrude "Extrude2'''''" add sketch "Sketch2 (3)" along normal blind 12 contours A1 L0 L1 L2 L3 L4 L6 L7 L9 | L1 L4 L5 L6 L8 L9 bodies 18 19 in component "screen-pms5003-joint"
extrude "Extrude3''''" cut 1 faces at (28.0085, 92.9303, 34.3885) along direction (0, 0, -1) blind 546 on bodies 18 bodies 18 in component "screen-pms5003-joint"
fillet "Fillet1'''" radius 3 1 edges at (31.3533, 95.2866, 28.3885) on bodies 18 in component "screen-pms5003-joint"
sketch "Sketch1 (5)" plane through (0, 0, 39.9885) normal (0, 0, 1) x (-1, 0, 0) in component "box"
  arc A0 (-28.8133, -30.5166) -> (-31.3533, -33.0566) centre (-28.8133, -33.0566) ccw
  line L0 (-31.3533, -33.0566) -> (-31.3533, -92.7466)
  arc A1 (-31.3533, -92.7466) -> (-28.8133, -95.2866) centre (-28.8133, -92.7466) ccw
  line L1 (-28.8133, -95.2866) -> (18.6847, -95.2866)
  arc A2 (18.6847, -95.2866) -> (21.2247, -92.7466) centre (18.6847, -92.7466) ccw
  line L2 (21.2247, -92.7466) -> (21.2247, -33.0566)
  arc A3 (21.2247, -33.0566) -> (18.6847, -30.5166) centre (18.6847, -33.0566) ccw
  line L3 (18.6847, -30.5166) -> (-28.8133, -30.5166)
  circle A4 centre (-28.8133, -33.0566) radius 1.27
  circle A5 centre (18.6847, -92.7466) radius 1.27
  circle A6 centre (-28.8133, -92.7466) radius 1.27
  circle A7 centre (18.6847, -33.0566) radius 1.27
  line L4 (-27.0533, -33.7866) -> (16.7467, -33.7866)
  line L5 (16.7467, -33.7866) -> (16.7467, -94.9866)
  line L6 (16.7467, -94.9866) -> (-27.0533, -94.9866)
  line L7 (-27.0533, -94.9866) -> (-27.0533, -33.7866)
  line L8 (16.2467, -34.2866) -> (-26.5533, -34.2866)
  line L9 (16.2467, -94.4866) -> (16.2467, -34.2866)
  line L10 (-26.5533, -94.4866) -> (16.2467, -94.4866)
  line L11 (-26.5533, -34.2866) -> (-26.5533, -94.4866)
  line L12 (-39.3533, -104.2866) -> (22.2247, -104.2866)
  line L13 (22.2247, -104.2866) -> (22.2247, -22.5166)
  line L14 (22.2247, -22.5166) -> (-39.3533, -22.5166)
  line L15 (-39.3533, -22.5166) -> (-39.3533, -104.2866)
  line L16 (-43.3533, -108.2866) -> (26.2247, -108.2866)
  line L17 (26.2247, -108.2866) -> (26.2247, -18.5166)
  line L18 (26.2247, -18.5166) -> (-43.3533, -18.5166)
  line L19 (-43.3533, -18.5166) -> (-43.3533, -108.2866)
  line L20 (-28.8843, -96.2866) -> (19.2157, -96.2866)
  point P0 (-26.5485, -34.2866)
  point P1 (-26.5533, -94.4836)
  point P2 (16.2824, -94.4866)
  point P3 (16.2467, -34.3194)
  dimension "d160" = 0.5
  dimension "d161" = 0.5
  dimension "d162" = 0.5
  dimension "d163" = 0.5
  dimension "d164" = 4
  dimension "d165" = 8
  dimension "d166" = 8
  dimension "d167" = 8
  dimension "d168" = 1
  constraint horizontal L4
  constraint vertical L5
  constraint horizontal L6
  constraint vertical L7
  constraint coincident P0 L8
  constraint coincident P3 L9
  constraint coincident P2 L10
  constraint coincident P1 L11
  constraint horizontal L12
  constraint vertical L13
  constraint horizontal L14
  constraint vertical L15
  measures "d160" distance of L7 L11
  measures "d161" distance of L4 L8
  measures "d162" distance of L5 L9
  measures "d163" distance of L6 L10
  measures "d165" distance of L3 L14
  measures "d166" distance of L12 L20
  measures "d167" distance of L0 L15
  measures "d168" distance of L2 L13
extrude "Extrude2''''''" add sketch "Sketch1 (5)" against normal blind 40 separate body contours L16 L17 L18 L19 makes body 20 in component "box"
extrude "Extrude1''''''" add sketch "Sketch1 (5)" along normal blind 4 contours A0 L0 A1 L1 A2 L2 A3 L3 | L12 L13 L14 L15 | L16 L17 L18 L19 bodies 20 in component "box"
fillet "Fillet1''''" radius 4 8 edges at (43.3533, 18.5166, 21.9885) (-26.2247, 18.5166, 21.9885) (43.3533, 108.2866, 21.9885) (-26.2247, 108.2866, 21.9885) (43.3533, 18.5166, 19.9885) (-26.2247, 18.5166, 19.9885) (43.3533, 108.2866, 19.9885) (-26.2247, 108.2866, 19.9885) on bodies 20 in component "box"
fillet "Fillet2" radius 3 4 edges at (39.3533, 22.5166, 19.9885) (-22.2247, 22.5166, 19.9885) (-22.2247, 104.2866, 19.9885) (39.3533, 104.2866, 19.9885) on bodies 20 in component "box"
sketch "Sketch2 (4)" plane through (0, 108.2866, 0) normal (0, 1, 0) x (-1, 0, 0) in component "box"
  line L0 (22.2247, -0.0115) -> (22.2247, 43.9885)
  line L1 (-39.3533, 43.9885) -> (-39.3533, -0.0115)
  line L2 (-39.3533, -0.0115) -> (22.2247, -0.0115)
  line L3 (22.2247, 43.9885) -> (-39.3533, 43.9885)
sketch "Sketch3 (2)" plane through (8.5643, 108.2866, 21.9885) normal (0, 1, 0) x (-1, 0, 0) in component "box"
  circle A0 centre (-7.32, -10.25) radius 10.5
  circle A1 centre (-7.32, -10.25) radius 9 construction
  line L0 (8.289, -16) -> (25.289, -16)
  line L1 (25.289, -16) -> (25.289, -20.5)
  line L2 (25.289, -20.5) -> (8.289, -20.5)
  line L3 (8.289, -20.5) -> (8.289, -16)
  line L4 (-30.789, -22) -> (30.789, -22)
  line L5 (30.789, -22) -> (30.789, 22)
  line L6 (-16.189, 18.4) -> (1.811, 18.4)
  line L7 (1.811, 18.4) -> (1.811, 12.7)
  line L8 (1.811, 12.7) -> (-16.189, 12.7)
  line L9 (-16.189, 12.7) -> (-16.189, 18.4)
  line L10 (-20.249, 16.4) -> (27.249, 16.4)
  line L11 (-0.189, 16.4) -> (-0.189, 14.7)
  line L12 (-0.189, 14.7) -> (-12.6931, 14.7)
  line L13 (-14.189, 16.4) -> (-14.189, 14.7)
  dimension "d181" = 21
  dimension "d182" = 1.5
  dimension "d183" = 5.5
  dimension "d184" = 17
  dimension "d185" = 4.5
  dimension "d198" = 2
  dimension "d199" = 2
  dimension "d200" = 2
  dimension "d201" = 2
  constraint concentric A0 A1
  constraint horizontal L0
  constraint vertical L1
  constraint horizontal L2
  constraint vertical L3
  constraint horizontal L6
  constraint vertical L7
  constraint horizontal L8
  constraint vertical L9
  measures "d181" diameter of A0
  measures "d182" distance of L2 L4
  measures "d183" distance of L1 L5
  measures "d184" distance of L0.start L0.end
  measures "d185" distance of L0.start L2.end
  measures "d198" distance of L6 L10
  measures "d199" distance of L7 L11
  measures "d200" distance of L8 L12
  measures "d201" distance of L9 L13
extrude "Extrude5''" cut sketch "Sketch3 (2)" against normal blind 4 bodies 20 in component "box"
extrude "Extrude3'''''" cut sketch "Sketch3 (2)" against normal blind 10 contours A0 | L0 L1 L2 L3 bodies 20 in component "box"
sketch "Sketch4" plane through (-26.2247, 0, 0) normal (-1, 0, 0) x (0, -1, 0) in component "box"
  line L0 (-104.2866, 43.9885) -> (-104.2866, -0.0115)
  line L1 (-104.2866, -0.0115) -> (-22.5166, -0.0115)
  line L2 (-22.5166, -0.0115) -> (-22.5166, 43.9885)
  line L3 (-22.5166, 43.9885) -> (-104.2866, 43.9885)
  line L4 (-52.0466, 32.3885) -> (-40.2466, 32.3885)
  line L5 (-40.2466, 32.3885) -> (-40.2466, 25.4385)
  line L6 (-40.2466, 25.4385) -> (-52.0466, 25.4385)
  line L7 (-52.0466, 25.4385) -> (-52.0466, 32.3885)
  line L8 (-60.6866, 29.0485) -> (-72.6866, 29.0485)
  line L9 (-72.6866, 29.0485) -> (-72.6866, 22.0485)
  line L10 (-72.6866, 22.0485) -> (-60.6866, 22.0485)
  line L11 (-60.6866, 22.0485) -> (-60.6866, 29.0485)
  line L12 (-70.6866, 24.0485) -> (-70.6866, 27.0485)
  line L13 (-70.6866, 27.0485) -> (-62.6866, 27.0485)
  line L14 (-62.6866, 24.0485) -> (-62.6866, 27.0485)
  line L15 (-70.6866, 24.0485) -> (-62.6866, 24.0485)
  line L16 (-42.2466, 27.4385) -> (-50.0466, 27.4385)
  line L17 (-42.2466, 29.3885) -> (-42.2466, 27.4385)
  line L18 (-50.0466, 29.3885) -> (-50.0466, 27.4385)
  line L19 (-43.2466, 30.3885) -> (-49.0466, 30.3885)
  dimension "d188" = 2
  dimension "d189" = 2
  dimension "d190" = 2
  dimension "d191" = 2
  dimension "d192" = 2
  dimension "d193" = 2
  dimension "d194" = 2
  dimension "d195" = 2
  constraint horizontal L4
  constraint vertical L5
  constraint horizontal L6
  constraint vertical L7
  constraint horizontal L8
  constraint vertical L9
  constraint horizontal L10
  constraint vertical L11
  measures "d188" distance of L9 L12
  measures "d189" distance of L8 L13
  measures "d190" distance of L11 L14
  measures "d191" distance of L10 L15
  measures "d192" distance of L6 L16
  measures "d193" distance of L5 L17
  measures "d194" distance of L7 L18
  measures "d195" distance of L4 L19
extrude "Extrude4''" cut sketch "Sketch4" against normal blind 4 contours L4 L5 L6 L7 | L8 L9 L10 L11 | L12 L13 L14 L15 bodies 20 in component "box"
sketch "Sketch5" plane through (43.3533, 0, 0) normal (1, 0, 0) x (0, 1, 0) in component "box"
  line L0 (104.2866, -0.0115) -> (104.2866, 43.9885)
  line L1 (104.2866, 43.9885) -> (22.5166, 43.9885)
  line L2 (22.5166, 43.9885) -> (22.5166, -0.0115)
  line L3 (22.5166, -0.0115) -> (104.2866, -0.0115)
  line L4 (32.5166, 33.9885) -> (32.5166, 9.9885)
  arc A0 (32.5166, 9.9885) -> (36.5166, 9.9885) centre (34.5166, 9.9885) ccw
  line L5 (36.5166, 9.9885) -> (36.5166, 33.9885)
  arc A1 (36.5166, 33.9885) -> (32.5166, 33.9885) centre (34.5166, 33.9885) ccw
  line L6 (34.5166, 33.9885) -> (34.5166, 9.9885) construction
  line L7 (51.9591, 9.9885) -> (51.9591, 33.9885)
  arc A2 (51.9591, 33.9885) -> (47.9591, 33.9885) centre (49.9591, 33.9885) ccw
  arc A3 (47.9591, 9.9885) -> (51.9591, 9.9885) centre (49.9591, 9.9885) ccw
  line L8 (47.9591, 33.9885) -> (47.9591, 9.9885)
  line L9 (67.4016, 9.9885) -> (67.4016, 33.9885)
  arc A4 (67.4016, 33.9885) -> (63.4016, 33.9885) centre (65.4016, 33.9885) ccw
  arc A5 (63.4016, 9.9885) -> (67.4016, 9.9885) centre (65.4016, 9.9885) ccw
  line L10 (63.4016, 33.9885) -> (63.4016, 9.9885)
  line L11 (82.8441, 9.9885) -> (82.8441, 33.9885)
  arc A6 (82.8441, 33.9885) -> (78.8441, 33.9885) centre (80.8441, 33.9885) ccw
  arc A7 (78.8441, 9.9885) -> (82.8441, 9.9885) centre (80.8441, 9.9885) ccw
  line L12 (78.8441, 33.9885) -> (78.8441, 9.9885)
  line L13 (98.2866, 9.9885) -> (98.2866, 33.9885)
  arc A8 (98.2866, 33.9885) -> (94.2866, 33.9885) centre (96.2866, 33.9885) ccw
  arc A9 (94.2866, 9.9885) -> (98.2866, 9.9885) centre (96.2866, 9.9885) ccw
  line L14 (94.2866, 33.9885) -> (94.2866, 9.9885)
  dimension "d204" = 10
  dimension "d205" = 10
  dimension "d206" = 4
  dimension "d207" = 10
  dimension "d210" = 61.77
  dimension "d211" = 0
  constraint tangent L4 A0
  constraint tangent A0 L5
  constraint parallel L4 L5
  constraint tangent L5 A1
  constraint tangent L4 A1
  constraint parallel L2 L6
  measures "d204" distance of L3 A0.centre
  measures "d205" distance of L1 A1.centre
  measures "d206" distance of L4 L5
  measures "d207" distance of L2 L4
extrude "Extrude6''" cut sketch "Sketch5" against normal blind 4 contours L4 A0 L5 A1 | L7 A2 A3 L8 | L9 A4 A5 L10 | L11 A6 A7 L12 | L13 A8 A9 L14 bodies 20 in component "box"
sketch "Sketch6 (2)" plane through (0, 18.5166, 0) normal (0, -1, 0) x (1, 0, 0) in component "box"
  line L0 (-22.2247, 43.9885) -> (-22.2247, -0.0115)
  line L1 (-22.2247, -0.0115) -> (39.3533, -0.0115)
  line L2 (39.3533, -0.0115) -> (39.3533, 43.9885)
  line L3 (39.3533, 43.9885) -> (-22.2247, 43.9885)
  line L4 (-12.2247, 33.9885) -> (-12.2247, 9.9885)
  arc A0 (-12.2247, 9.9885) -> (-8.2247, 9.9885) centre (-10.2247, 9.9885) ccw
  line L5 (-8.2247, 9.9885) -> (-8.2247, 33.9885)
  arc A1 (-8.2247, 33.9885) -> (-12.2247, 33.9885) centre (-10.2247, 33.9885) ccw
  line L6 (-10.2247, 33.9885) -> (-10.2247, 9.9885) construction
  line L7 (1.6319, 33.9885) -> (1.6319, 9.9885)
  arc A2 (1.6319, 9.9885) -> (5.6319, 9.9885) centre (3.6319, 9.9885) ccw
  arc A3 (5.6319, 33.9885) -> (1.6319, 33.9885) centre (3.6319, 33.9885) ccw
  line L8 (5.6319, 9.9885) -> (5.6319, 33.9885)
  line L9 (15.4886, 33.9885) -> (15.4886, 9.9885)
  arc A4 (15.4886, 9.9885) -> (19.4886, 9.9885) centre (17.4886, 9.9885) ccw
  arc A5 (19.4886, 33.9885) -> (15.4886, 33.9885) centre (17.4886, 33.9885) ccw
  line L10 (19.4886, 9.9885) -> (19.4886, 33.9885)
  line L11 (29.3453, 33.9885) -> (29.3453, 9.9885)
  arc A6 (29.3453, 9.9885) -> (33.3453, 9.9885) centre (31.3453, 9.9885) ccw
  arc A7 (33.3453, 33.9885) -> (29.3453, 33.9885) centre (31.3453, 33.9885) ccw
  line L12 (33.3453, 9.9885) -> (33.3453, 33.9885)
  dimension "d214" = 10
  dimension "d216" = 10
  dimension "d217" = 4
  dimension "d220" = 41.57
  dimension "d221" = 0
  dimension "d235" = 10
  constraint tangent L4 A0
  constraint tangent A0 L5
  constraint parallel L4 L5
  constraint tangent L5 A1
  constraint tangent L4 A1
  constraint vertical L6
  measures "d214" distance of L1 A0.centre
  measures "d216" distance of L0 L4
  measures "d217" distance of L4 L5
  measures "d235" distance of L3 A1.centre
extrude "Extrude7''" cut sketch "Sketch6 (2)" against normal blind 5 contours L4 A0 L5 A1 | L7 A2 A3 L8 | L9 A4 A5 L10 | L11 A6 A7 L12 bodies 20 in component "box"
extrude "Extrude8'" add 1 faces at (42.0199, 50.7733, -0.0115) along direction (0, 0, -1) blind 6 on bodies 20 bodies 20 in component "box"
sketch "Sketch1 (6)" plane through (0, 0, -6.0115) normal (0, 0, -1) x (1, 0, 0) in component "top"
  arc A0 (-26.2247, -104.2866) -> (-22.2247, -108.2866) centre (-22.2247, -104.2866) ccw
  line L0 (-22.2247, -108.2866) -> (39.3533, -108.2866)
  arc A1 (39.3533, -108.2866) -> (43.3533, -104.2866) centre (39.3533, -104.2866) ccw
  line L1 (43.3533, -104.2866) -> (43.3533, -22.5166)
  arc A2 (43.3533, -22.5166) -> (39.3533, -18.5166) centre (39.3533, -22.5166) ccw
  line L2 (39.3533, -18.5166) -> (-22.2247, -18.5166)
  arc A3 (-22.2247, -18.5166) -> (-26.2247, -22.5166) centre (-22.2247, -22.5166) ccw
  line L3 (-26.2247, -22.5166) -> (-26.2247, -104.2866)
  line L4 (39.3533, -25.5166) -> (39.3533, -101.2866)
  arc A4 (36.3533, -104.2866) -> (39.3533, -101.2866) centre (36.3533, -101.2866) ccw
  line L5 (36.3533, -104.2866) -> (-19.2247, -104.2866)
  arc A5 (-22.2247, -101.2866) -> (-19.2247, -104.2866) centre (-19.2247, -101.2866) ccw
  line L6 (-22.2247, -101.2866) -> (-22.2247, -25.5166)
  arc A6 (-19.2247, -22.5166) -> (-22.2247, -25.5166) centre (-19.2247, -25.5166) ccw
  line L7 (-19.2247, -22.5166) -> (36.3533, -22.5166)
  arc A7 (39.3533, -25.5166) -> (36.3533, -22.5166) centre (36.3533, -25.5166) ccw
  arc A8 (38.8533, -25.5166) -> (36.3533, -23.0166) centre (36.3533, -25.5166) ccw
  line L8 (-19.2247, -23.0166) -> (36.3533, -23.0166)
  arc A9 (-19.2247, -23.0166) -> (-21.7247, -25.5166) centre (-19.2247, -25.5166) ccw
  line L9 (-21.7247, -101.2866) -> (-21.7247, -25.5166)
  arc A10 (-21.7247, -101.2866) -> (-19.2247, -103.7866) centre (-19.2247, -101.2866) ccw
  line L10 (36.3533, -103.7866) -> (-19.2247, -103.7866)
  arc A11 (36.3533, -103.7866) -> (38.8533, -101.2866) centre (36.3533, -101.2866) ccw
  line L11 (38.8533, -25.5166) -> (38.8533, -101.2866)
  dimension "d226" = 0.5